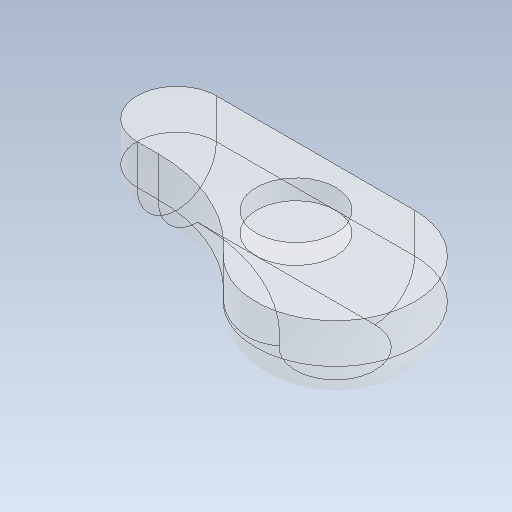
# Autodesk Inventor part: cauciuc ochelari
Saved by Autodesk Inventor 2020 (Build 240168000, 168)
## iProperties
Created: 2019-12-05
Part Number: cauciuc ochelari
Material: Rubber, Silicone
Document SubType Name: Modeling
Designer: Bianca
Density: 1.25 g/cm^3
Appearance: Rubber - Black
Mass: 0.00592847 g
Surface Area: 0.194037 cm^2
Volume: 0.00474278 cm^3
Author: Bianca
Autodesk Inventor part; units mm, degrees
ref_plane "YZ Plane" through (0, 0, 0) normal (1, 0, 0) x (0, 1, 0)
ref_plane "XZ Plane" through (0, 0, 0) normal (0, 1, 0) x (-1, 0, 0)
ref_plane "XY Plane" through (0, 0, 0) normal (0, 0, 1) x (1, 0, 0)
sketch "Sketch1" plane through (0, 0, 0) normal (0, 1, 0) x (-1, 0, 0)
  line L0 (1, 0) -> (4, 0) construction
  line L1 (4, 0) -> (4, -1.5) construction
  line L2 (3.5, -2) -> (1, -2)
  line L3 (0, -1) -> (0, -1)
  arc A0 (1, 0) -> (0, -1) centre (1, -1) ccw
  arc A1 (0, -1) -> (1, -2) centre (1, -1) ccw
  arc A2 (3.5, -2) -> (4, -1.5) centre (3.5, -1.5) ccw
  arc A3 (1.7454, -0.3333) -> (1, -2) centre (1, -1) ccw
  arc A4 (3.5, -2) -> (3.5, -1) centre (3.5, -1.5) ccw
  line L4 (3.5, -1) -> (3.2361, -1)
  arc A5 (1.7454, -0.3333) -> (3.2361, -1) centre (3.2361, 1) ccw
  point P0 (0, 0)
  point P1 (4, -2)
  point P2 (0, -2)
  point P3 (2, -1)
  dimension "d0" = 4
  dimension "d1" = 2
  dimension "d2" = 1
  dimension "d3" = 0.5
  dimension "d4" = 2
  constraints: 13 point on circle, 10 end point, 9 tangent, 7 point on line, 6 centre point, 3 concentric, 2 coincident, 2 horizontal, 2 parallel, 1 perpendicular
  measures "d0" distance of point (4, -2) point (0, -2)
  measures "d1" distance of L0.end point (4, -2)
  measures "d2" radius of A0
  measures "d3" radius of A2
  measures "d4" radius of A5
extrude "Extrusion1" add sketch "Sketch1" along normal blind 1
sketch "Sketch2" plane through (0, 1, 0) normal (0, 1, 0) x (1, 0, 0)
  circle A0 centre (-1.7477, 1.2518) radius 0.5
  point P0 (0, 0)
  dimension "d7" = 1
  constraints: 1 centre point
  measures "d7" diameter of A0
hole "Hole1" at (-1.7477, 1, -1.2518) direction (0, -1, 0) diameter 1 depth 0.25
fillet "Fillet2" radius 0.5 5 edges at (-0.0871, 0, -0.5918) (-2.25, 0, -2) (-4, 0, -1.5) (-3.368, 0, -1) (-2.4196, 0, -0.8257)
body "Solid1"
